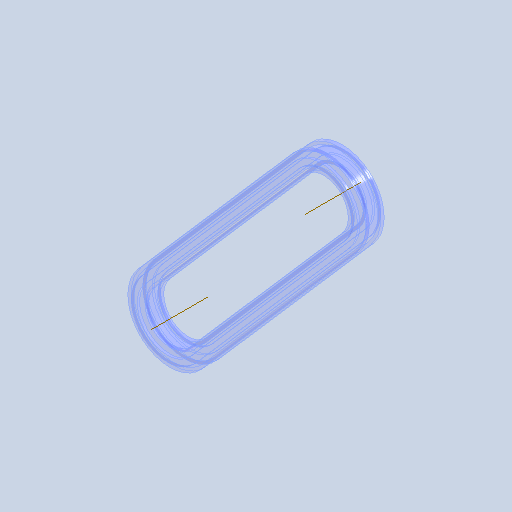
# Autodesk Inventor part: Cadena de rodillos
Saved by Autodesk Inventor 2022.1 (Build 261234000, 234)
## iProperties
Created: 2021-09-12
Part Number: Cadena de rodillos
Material: Generic
Document SubType Name: Modeling
Designer: seb_0
Density: 1 g/cm^3
Appearance: Clear - Blue
CustomPartVersion: 1
Author: seb_0
Autodesk Inventor part; units mm, degrees
ref_plane "YZ Plane" through (0, 0, 0) normal (1, 0, 0) x (0, 1, 0)
ref_plane "XZ Plane" through (0, 0, 0) normal (0, 1, 0) x (-1, 0, 0)
ref_plane "XY Plane" through (0, 0, 0) normal (0, 0, 1) x (1, 0, 0)
ref_plane "Plano de trabajo2" through (0, 0, 0) normal (-1, 0, 0) x (0, 0, 1)
ref_plane "Plano de trabajo3" through (130.2876, 149.6223, 0) normal (-0.959493, -0.2817326, 0) x (0, 0, 1)
sketch "Trayectoria" plane through (0, 0, 0) normal (0, 0, 1) x (1, 0, 0)
  arc A0 (-21.2474, 18.5018) -> (21.2474, -18.5018) centre (0, 0) ccw
  arc A1 (151.535, 131.1205) -> (109.0402, 168.124) centre (130.2876, 149.6223) ccw
  line L0 (151.535, 131.1205) -> (21.2474, -18.5018)
  line L1 (-21.2474, 18.5018) -> (109.0402, 168.124)
  dimension "d31" = 14.73
  constraints: 4 end point, 4 point on circle, 2 centre point
ref_plane "Plano de sección" through (21.2474, -18.5018, 0) normal (0.6566988, 0.754153, 0) x (0, 0, 1)
sketch "Boceto de sección" plane through (21.2474, -18.5018, 0) normal (0.6566988, 0.754153, 0) x (0, 0, 1)
  line L0 (-9.8, -2.54) -> (9.8, -2.54)
  line L1 (9.8, -2.54) -> (9.8, 2.54)
  line L2 (9.8, 2.54) -> (-9.8, 2.54)
  line L3 (-9.8, 2.54) -> (-9.8, -2.54)
  line L4 (-4.825, -5.08) -> (4.825, -5.08)
  line L5 (4.825, -5.08) -> (4.825, 5.08)
  line L6 (4.825, 5.08) -> (-4.825, 5.08)
  line L7 (-4.825, 5.08) -> (-4.825, -5.08)
  line L8 (-4.825, 0) -> (4.825, 0) construction
  line L9 (-7.825, -7.365) -> (-4.825, -7.365)
  line L10 (-4.825, -7.365) -> (-4.825, 7.365)
  line L11 (-4.825, 7.365) -> (-7.825, 7.365)
  line L12 (-7.825, 7.365) -> (-7.825, -7.365)
  line L13 (4.825, -7.365) -> (7.825, -7.365)
  line L14 (7.825, -7.365) -> (7.825, 7.365)
  line L15 (7.825, 7.365) -> (4.825, 7.365)
  line L16 (4.825, 7.365) -> (4.825, -7.365)
  line L17 (-9.8, 0) -> (9.8, 0) construction
  point P0 (0, 0)
  point P1 (0, 0)
  dimension "d21" = 5.08
  dimension "d22" = 10.16
  dimension "d23" = 9.65
  dimension "d24" = 3
  dimension "d31" = 14.73
  dimension "d32" = 19.6
  constraints: 36 end point, 8 midpoint, 8 parallel, 4 horizontal, 4 perpendicular, 3 collinear, 1 coincident, 1 other
  measures "d21" distance between parallel lines of L2 L0
  measures "d22" distance between parallel lines of L6 L4
  measures "d23" distance between parallel lines of L5 L7
  measures "d24" distance between parallel lines of L12 L10
  measures "d31" distance between parallel lines of L11 L9
  measures "d32" distance between parallel lines of L1 L3
sweep "Sólido" add profiles "Boceto de sección" path "Trayectoria" path curves L1 A1 L0 A0
pattern_of_one "Strand Pattern"
equation "\"d21\" = da_d2"
equation "\"d22\" = da_d1"
equation "\"d23\" = da_b1"
equation "\"d24\" = da_t1 + da_t2"
equation "\"d30\" = da_pt"
equation "\"da_p\" = 15.875"
equation "\"da_b1\" = 9.65"
equation "\"da_h2\" = 14.73"
equation "\"da_h3\" = 13.72"
equation "\"da_d1\" = 10.16"
equation "\"da_d2\" = 5.08"
equation "\"da_pt\" = 16.59"
equation "\"da_b\" = 19.6"
equation "\"da_t1\" = 1.5"
equation "\"da_t2\" = 1.5"
body "Solid1"
